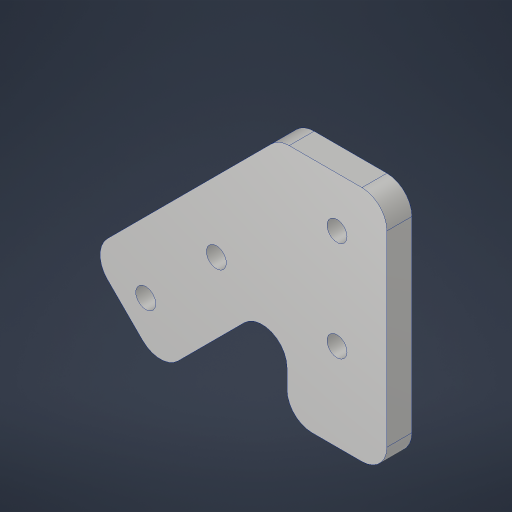
# Autodesk Inventor part: CL4-008
Saved by Autodesk Inventor 2023.4 (Build 274418000, 418)
## iProperties
Created: 2025-02-04
Part Number: CL4-008
Material: Aluminum 6061
Document SubType Name: Modeling
Designer: brand
Density: 2.7 g/cm^3
Appearance: Aluminum - Flat
Author: brand
Autodesk Inventor part; units mm, degrees
ref_plane "YZ Plane" through (0, 0, 0) normal (1, 0, 0) x (0, 1, 0)
ref_plane "XZ Plane" through (0, 0, 0) normal (0, 1, 0) x (-1, 0, 0)
ref_plane "XY Plane" through (0, 0, 0) normal (0, 0, 1) x (1, 0, 0)
sketch "Sketch1" plane through (0, 0, 0) normal (0, 0, 1) x (1, 0, 0)
  line L0 (0, 0) -> (0, -57.15) construction
  line L1 (0, 0) -> (-53.8815, -53.8815) construction
  line L2 (12.7, 3.175) -> (-14.7855, 3.175)
  line L3 (-14.7855, 3.175) -> (-62.8618, -44.9013)
  line L4 (-62.8618, -44.9013) -> (-44.9013, -62.8618)
  line L5 (-44.9013, -62.8618) -> (-12.7, -30.6605)
  line L6 (-12.7, -30.6605) -> (-12.7, -57.15)
  line L7 (-12.7, -57.15) -> (12.7, -57.15)
  line L8 (12.7, -57.15) -> (12.7, 3.175)
  dimension "d0" = 45
  dimension "d1" = 57.15
  dimension "d2" = 76.2
  dimension "d3" = 3.175
  dimension "d4" = 25.4
  dimension "d5" = 25.4
  constraints: 19 end point, 6 perpendicular, 2 midpoint, 1 horizontal, 1 vertical
  measures "d0" angle of L0 L1
  measures "d1" distance of L0.end L0.start
  measures "d2" distance of L1.end L0.start
  measures "d3" distance from line of L2 L0.start
  measures "d4" distance of L6.end L7.end
  measures "d5" distance of L3.end L4.end
extrude "Extrusion1" add sketch "Sketch1" against normal blind 6.35
sketch "Sketch2" plane through (0, 0, 0) normal (0, 0, 1) x (1, 0, 0)
  line L0 (-44.9013, -62.8618) -> (-62.8618, -44.9013) construction
  line L1 (-62.8618, -44.9013) -> (-14.7855, 3.175) construction
  line L2 (-14.7855, 3.175) -> (12.7, 3.175) construction
  line L3 (12.7, 3.175) -> (12.7, -57.15) construction
  line L4 (12.7, -57.15) -> (-12.7, -57.15) construction
  line L5 (-12.7, -57.15) -> (-12.7, -30.6605) construction
  line L6 (-12.7, -30.6605) -> (-44.9013, -62.8618) construction
  line L7 (-44.9013, -62.8618) -> (-62.8618, -44.9013) construction
  line L8 (-62.8618, -44.9013) -> (-14.7855, 3.175) construction
  line L9 (-14.7855, 3.175) -> (12.7, 3.175) construction
  line L10 (12.7, 3.175) -> (12.7, -57.15) construction
  line L11 (12.7, -57.15) -> (-12.7, -57.15) construction
  line L12 (-12.7, -57.15) -> (-12.7, -30.6605) construction
  line L13 (-12.7, -30.6605) -> (-44.9013, -62.8618) construction
  line L14 (0, 0) -> (0, -57.15) construction
  line L15 (12.7, -57.15) -> (-12.7, -57.15) construction
  line L16 (0, 0) -> (-53.8815, -53.8815) construction
  line L17 (-44.9013, -62.8618) -> (-62.8618, -44.9013) construction
  line L18 (-12.7, -30.6605) -> (-12.7, 3.175) construction
  line L19 (-14.7855, 3.175) -> (12.7, 3.175) construction
  point P0 (-30.6605, -30.6605)
  point P1 (-48.621, -48.621)
  point P2 (0, -9.525)
  point P3 (0, -34.925)
  point P4 (-12.7, -12.7)
  point P5 (-12.7, -13.7428)
  dimension "d8" = 25.4
  dimension "d9" = 25.4
  dimension "d19" = 12.7
  dimension "d21" = 25.4
  constraints: 7 point on line, 6 end point, 4 midpoint, 1 vertical
  measures "d8" distance of point (-48.621, -48.621) point (-30.661, -30.661)
  measures "d9" distance of point (0, -9.525) point (0, -34.925)
  measures "d19" distance from line of point (0, -9.525) L2
  measures "d21" distance of point (-30.661, -30.661) point (-12.7, -12.7)
hole "Hole1" at (-30.6605, -30.6605, 0) at (-48.621, -48.621, 0) at (0, -9.525, 0) at (0, -34.925, 0) direction (0, 0, -1) diameter 5.1054 end through all clearance for "Flat Head Machine Screw (82)" size "#10" standard "Ansi Unified Screw Threads"
fillet "Fillet1" radius 6.35 7 edges at (12.7, 3.175, -3.175) (-14.7855, 3.175, -3.175) (-62.8618, -44.9013, -3.175) (-44.9013, -62.8618, -3.175) (-12.7, -30.6605, -3.175) (-12.7, -57.15, -3.175) (12.7, -57.15, -3.175)
equation "\"d5\" = d4"
body "Solid1"
